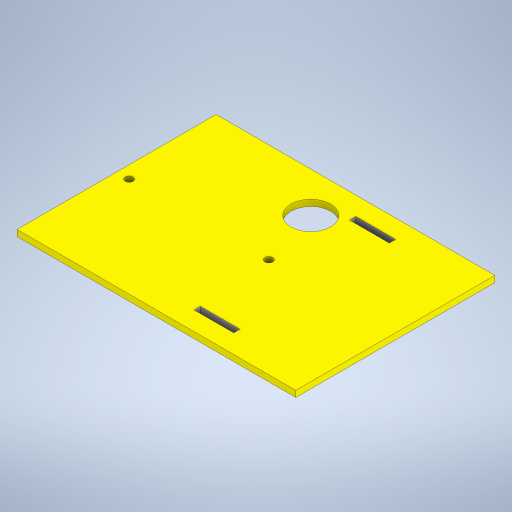
# Autodesk Inventor part: Base
Saved by Autodesk Inventor 2024 (Build 280153000, 153)
## iProperties
Created: 2024-04-22
Part Number: Base
Material: Generic
Document SubType Name: Modeling
Designer: samue
Density: 1 g/cm^3
Appearance: Default
Author: samue
Autodesk Inventor part; units mm, degrees
ref_plane "YZ Plane" through (0, 0, 0) normal (1, 0, 0) x (0, 1, 0)
ref_plane "XZ Plane" through (0, 0, 0) normal (0, 1, 0) x (-1, 0, 0)
ref_plane "XY Plane" through (0, 0, 0) normal (0, 0, 1) x (1, 0, 0)
sketch "Sketch1" plane through (0, 0, 0) normal (0, 1, 0) x (-1, 0, 0)
  line L0 (70, 50) -> (-70, 50)
  line L1 (-70, 50) -> (-70, -50)
  line L2 (-70, -50) -> (70, -50)
  line L3 (70, -50) -> (70, 50)
  line L4 (70, 50) -> (-70, -50) construction
  line L5 (-70, 50) -> (70, -50) construction
  point P0 (0, 0)
  dimension "d0" = 140
  dimension "d1" = 100
  constraints: 12 end point, 2 midpoint, 2 parallel, 1 horizontal, 1 perpendicular
  measures "d0" distance of L2.end L1.end
  measures "d1" distance of L0.end L1.end
extrude "Extrusion1" add sketch "Sketch1" along normal blind 3.125
sketch "Sketch9" plane through (0, 3.125, 0) normal (0, 1, 0) x (1, 0, 0)
  circle A0 centre (-2.2797, 29.8308) radius 10
  point P0 (0, 0)
  dimension "d41" = 20
  constraints: 1 centre point
  measures "d41" diameter of A0
extrude "Extrusion9" cut sketch "Sketch9" against normal blind 10
sketch "Sketch10" plane through (0, 3.125, 0) normal (0, 1, 0) x (1, 0, 0)
  circle A0 centre (-63.7193, 0) radius 2
  point P0 (0, 0)
  dimension "d44" = 4
  constraints: 1 centre point
  measures "d44" diameter of A0
extrude "Extrusion10" cut sketch "Sketch10" against normal blind 5
sketch "Sketch11" plane through (0, 3.125, 0) normal (0, 1, 0) x (1, 0, 0)
  circle A0 centre (6.4375, 0) radius 2
  point P0 (0, 0)
  dimension "d47" = 4
  constraints: 1 centre point
  measures "d47" diameter of A0
extrude "Extrusion11" cut sketch "Sketch11" against normal blind 5
sketch "Sketch12" plane through (0, 3.125, 0) normal (0, 1, 0) x (1, 0, 0)
  point P0 (0, 0)
sketch "Sketch14" plane through (0, 3.125, 0) normal (0, 1, 0) x (1, 0, 0)
  line L0 (9.4435, 40.7) -> (29.4435, 40.7)
  line L1 (29.4435, 40.7) -> (29.4435, 37.545)
  line L2 (29.4435, 37.545) -> (9.4435, 37.545)
  line L3 (9.4435, 37.545) -> (9.4435, 40.7)
  line L4 (9.4435, 40.7) -> (29.4435, 37.545) construction
  line L5 (29.4435, 40.7) -> (9.4435, 37.545) construction
  line L6 (9.4435, -37.455) -> (29.4435, -37.455)
  line L7 (29.4435, -37.455) -> (29.4435, -40.61)
  line L8 (29.4435, -40.61) -> (9.4435, -40.61)
  line L9 (9.4435, -40.61) -> (9.4435, -37.455)
  line L10 (9.4435, -37.455) -> (29.4435, -40.61) construction
  line L11 (29.4435, -37.455) -> (9.4435, -40.61) construction
  line L12 (70, 50) -> (-70, 50) projected
  point P0 (0, 0)
  point P1 (19.4435, 39.1225)
  point P2 (19.4435, -39.0325)
  dimension "d60" = 20
  dimension "d61" = 3.155
  dimension "d62" = 20
  dimension "d63" = 3.155
  dimension "d64" = 75
  dimension "d67" = 9.3
  constraints: 24 end point, 4 midpoint, 4 parallel, 2 horizontal, 2 perpendicular, 1 vertical alignment
  measures "d60" distance of L1.end L2.end
  measures "d61" distance of L0.end L1.end
  measures "d62" distance of L7.end L8.end
  measures "d63" distance of L6.end L7.end
  measures "d64" distance between parallel lines of L6 L2
  measures "d67" distance between parallel lines of L12 L0
extrude "Extrusion13" cut sketch "Sketch14" against normal blind 3.125
body "Solid1"
